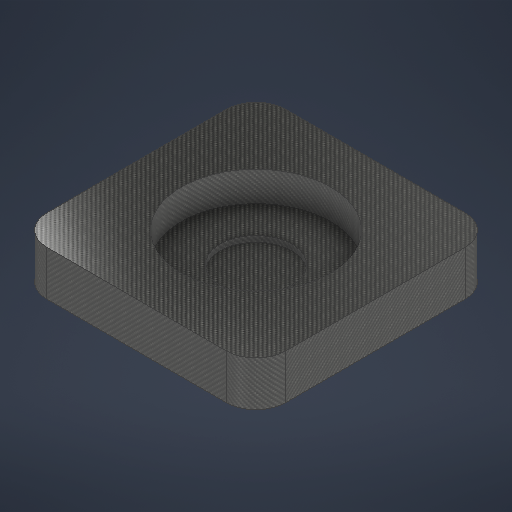
# Autodesk Inventor part: HANDBASE2
Saved by Autodesk Inventor 2027.1 (Build 311270010, 270A)
## iProperties
Created: 2026-08-27
Part Number: HANDBASE2
Material: Generic
Document SubType Name: Modeling
Designer: RIDDHIMAN
Density: 1 g/cm^3
Appearance: Default
Author: RIDDHIMAN
Autodesk Inventor part; units mm, degrees
ref_plane "YZ Plane" through (0, 0, 0) normal (1, 0, 0) x (0, 1, 0)
ref_plane "XZ Plane" through (0, 0, 0) normal (0, 1, 0) x (-1, 0, 0)
ref_plane "XY Plane" through (0, 0, 0) normal (0, 0, 1) x (1, 0, 0)
sketch "Sketch1" plane through (0, 0, 0) normal (0, 1, 0) x (-1, 0, 0)
  line L0 (125, 125) -> (-125, 125)
  line L1 (-125, 125) -> (-125, -125)
  line L2 (-125, -125) -> (125, -125)
  line L3 (125, -125) -> (125, 125)
  line L4 (125, 125) -> (-125, -125) construction
  line L5 (-125, 125) -> (125, -125) construction
  line L6 (-200, -200) -> (200, -200)
  line L7 (200, -200) -> (200, 200)
  line L8 (200, 200) -> (-200, 200)
  line L9 (-200, 200) -> (-200, -200)
  line L10 (-200, -200) -> (200, 200) construction
  line L11 (200, -200) -> (-200, 200) construction
  point P0 (0, 0)
  dimension "d0" = 250
  dimension "d1" = 250
  dimension "d2" = 400
  dimension "d3" = 400
  constraints: 24 end point, 4 midpoint, 4 parallel, 2 horizontal, 2 perpendicular
  measures "d0" distance of L2.end L1.end
  measures "d1" distance of L1.end L0.end
  measures "d2" distance of L8.end L7.end
  measures "d3" distance of L7.end L6.end
extrude "Extrusion1" add sketch "Sketch1" along normal blind 75
sketch "Sketch2" plane through (0, 0, 0) normal (0, -1, 0) x (1, 0, 0)
  line L0 (-125, -125) -> (125, -125) projected
  line L1 (125, 125) -> (-125, 125)
  line L2 (-125, 125) -> (-125, -125)
  line L3 (-125, -125) -> (125, -125)
  line L4 (125, -125) -> (125, 125)
  line L5 (125, 125) -> (-125, -125) construction
  line L6 (-125, 125) -> (125, -125) construction
  point P0 (0, 0)
  constraints: 12 end point, 2 midpoint, 2 parallel, 1 horizontal, 1 perpendicular
extrude "Extrusion2" add sketch "Sketch2" against normal blind 25
fillet "Fillet1" radius 50 4 edges at (200, 37.5, -200) (200, 37.5, 200) (-200, 37.5, -200) (-200, 37.5, 200)
sketch "Sketch3" plane through (0, 0, 0) normal (0, -1, 0) x (1, 0, 0)
  circle A0 centre (150, -150) radius 22.5
  arc A1 (150, -200) -> (200, -150) centre (150, -150) ccw projected
  circle A2 centre (-150, -150) radius 22.5
  circle A3 centre (-150, 150) radius 22.5
  circle A4 centre (150, 150) radius 22.5
  arc A5 (-200, -150) -> (-150, -200) centre (-150, -150) ccw projected
  arc A6 (-150, 200) -> (-200, 150) centre (-150, 150) ccw projected
  arc A7 (200, 150) -> (150, 200) centre (150, 150) ccw projected
  point P0 (0, 0)
  dimension "d9" = 45
  dimension "d10" = 45
  dimension "d11" = 45
  dimension "d12" = 45
  constraints: 4 centre point, 4 concentric
  measures "d9" diameter of A0
  measures "d10" diameter of A2
  measures "d11" diameter of A3
  measures "d12" diameter of A4
extrude "Extrusion3" cut sketch "Sketch3" against normal blind 25
fillet "Fillet2" radius 125 4 edges at (-125, 50, -125) (-125, 50, 125) (125, 50, -125) (125, 50, 125)
sketch "Sketch4" plane through (0, 25, 0) normal (0, 1, 0) x (1, 0, 0)
  circle A0 centre (0, 0) radius 60
  dimension "d16" = 120
  constraints: 1 centre point, 1 coincident
  measures "d16" diameter of A0
extrude "Extrusion4" cut sketch "Sketch4" against normal blind 10
body "Solid1"
